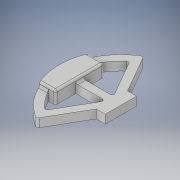
# Autodesk Inventor part: pieceMere
Saved by Autodesk Inventor 2019 (Build 230136000, 136)
## iProperties
Created: 2021-01-08
Part Number: pieceMere
Material: Générique
Document SubType Name: Modeling
Designer: tom.mousset
Density: 1 g/cm^3
Appearance: Par défaut
Author: tom.mousset
Autodesk Inventor part; units mm, degrees
ref_plane "YZ Plane" through (0, 0, 0) normal (1, 0, 0) x (0, 1, 0)
ref_plane "XZ Plane" through (0, 0, 0) normal (0, 1, 0) x (-1, 0, 0)
ref_plane "XY Plane" through (0, 0, 0) normal (0, 0, 1) x (1, 0, 0)
sketch "Esquisse1" plane through (0, 0, 0) normal (0, 1, 0) x (-1, 0, 0)
  circle A0 centre (0, 0) radius 80 construction
  line L0 (0, 0) -> (40, 69.282) construction
  line L1 (0, 0) -> (40, -69.282) construction
  line L2 (0, 0) -> (26.8174, 0)
  line L3 (78.7655, 14) -> (78.7655, 26) construction
  line L4 (78.7655, 26) -> (57.7655, 26) construction
  line L5 (57.7655, 26) -> (57.7655, 14) construction
  line L6 (57.7655, 14) -> (78.7655, 14) construction
  line L7 (78.7655, -14) -> (78.7655, -26) construction
  line L8 (78.7655, -26) -> (57.7655, -26) construction
  line L9 (57.7655, -26) -> (57.7655, -14) construction
  line L10 (57.7655, -14) -> (78.7655, -14) construction
  arc A1 (40, -69.282) -> (40, 69.282) centre (0, 0) ccw construction
  arc A2 (39.5, -68.416) -> (39.5, 68.416) centre (0, 0) ccw construction
  line L11 (0, 20) -> (0, -20)
  line L12 (0, 20) -> (11.547, 20)
  line L13 (0, -20) -> (11.547, -20)
  line L14 (47.8425, -62.8657) -> (11.547, 0) construction
  line L15 (11.547, 0) -> (47.8425, 62.8657) construction
  arc A3 (42.796, -54.1249) -> (42.796, 54.1249) centre (0, 0) ccw construction
  line L16 (61.6441, -31) -> (52.7655, -31)
  line L17 (52.7655, -31) -> (52.7655, -5)
  line L18 (52.7655, 5) -> (52.7655, 31)
  line L19 (52.7655, 31) -> (61.6441, 31)
  arc A4 (67.5648, 14) -> (63.914, 26) centre (0, 0) ccw construction
  arc A5 (63.914, -26) -> (67.5648, -14) centre (0, 0) ccw construction
  arc A6 (42.796, -54.1249) -> (61.6441, -31) centre (0, 0) ccw
  arc A7 (61.6441, 31) -> (42.796, 54.1249) centre (0, 0) ccw
  line L20 (42.796, 54.1249) -> (14.4338, 5)
  line L21 (14.4338, -5) -> (42.796, -54.1249)
  line L22 (52.7655, 5) -> (14.4338, 5)
  line L23 (52.7655, -5) -> (14.4338, -5)
  line L24 (11.547, -20) -> (39.5, -68.416)
  line L25 (11.547, 20) -> (39.5, 68.416)
  arc A8 (74.5989, 26) -> (39.5, 68.416) centre (0, 0) ccw
  arc A9 (77.7496, -14) -> (77.7496, 14) centre (0, 0) ccw
  arc A10 (39.5, -68.416) -> (74.5989, -26) centre (0, 0) ccw
  line L26 (74.5989, -26) -> (57.7655, -26)
  line L27 (57.7655, -14) -> (57.7655, -26)
  line L28 (57.7655, -14) -> (77.7496, -14)
  line L29 (74.5989, 26) -> (57.7655, 26)
  line L30 (57.7655, 26) -> (57.7655, 14)
  line L31 (57.7655, 14) -> (77.7496, 14)
  dimension "d10" = 79
  dimension "d0" = 160
  dimension "d1" = 60
  dimension "d2" = 60
  dimension "d3" = 12
  dimension "d4" = 21
  dimension "d5" = 14
  dimension "d6" = 12
  dimension "d7" = 14
  dimension "d8" = 21
  dimension "d9" = 80
  dimension "d11" = 40
  dimension "d12" = 20
  dimension "d13" = 10
  dimension "d14" = 10
  dimension "d15" = 69
  dimension "d16" = 5
  dimension "d17" = 5
  dimension "d20" = 5
  dimension "d21" = 5
  constraints: 64 end point, 28 point on circle, 17 point on line, 10 centre point, 10 coincident, 9 perpendicular, 8 parallel, 5 collinear, 3 horizontal, 2 vertical, 1 concentric, 11 other
  measures "d0" diameter of A0
  measures "d1" angle of L2 L1
  measures "d2" angle of L2 L0
  measures "d3" distance of L3.start L3.end
  measures "d4" distance of L4.end L3.end
  measures "d5" distance from line of L2.end L6
  measures "d6" distance of L7.start L7.end
  measures "d7" vertical distance of L2.end L7.start
  measures "d8" distance of L7.end L8.end
  measures "d9" radius of A1
  measures "d11" distance of L11.start L11.end
  measures "d12" distance of point (0, 0) L11.start
  measures "d13" distance between parallel lines of L0 L15
  measures "d14" distance between parallel lines of L1 L14
  measures "d15" radius of A3
  measures "d16" distance between parallel lines of L16 L8
  measures "d17" distance between parallel lines of L17 L9
  measures "d20" distance between parallel lines of L5 L18
  measures "d21" distance between parallel lines of L4 L19
extrude "Extrusion1" add sketch "Esquisse1" along normal blind 11
sketch "Esquisse2" plane through (0, 11, 0) normal (0, 1, 0) x (1, 0, 0)
  circle A0 centre (0, 0) radius 79 construction
  line L0 (-52.7655, 31) -> (-61.6441, 31) construction
  line L1 (-61.6441, -31) -> (-52.7655, -31) construction
  line L2 (-52.7655, 31) -> (-52.7655, -31)
  arc A1 (-39.5, 68.416) -> (-74.5989, 26) centre (0, 0) ccw construction
  arc A2 (-74.5989, -26) -> (-39.5, -68.416) centre (0, 0) ccw construction
  arc A3 (-72.6636, 31) -> (-72.6636, -31) centre (0, 0) ccw
  line L3 (-52.7655, 31) -> (-72.6636, 31)
  line L4 (-72.6636, -31) -> (-52.7655, -31)
  constraints: 6 end point, 5 point on circle, 2 centre point, 2 coincident, 2 collinear, 1 perpendicular
extrude "Extrusion2" add sketch "Esquisse2" along normal blind 5
fillet "Congé1" radius 2.5 16 edges at (-67.1539, 11, -31) (-67.1539, 11, 31) (-52.7655, 11, 0) (-62.7145, 16, -31) (-52.7655, 16, 0) (-62.7145, 16, 31) (-52.7655, 5.5, 31) (-52.7655, 13.5, 31) (-52.7655, 5.5, -31) (-52.7655, 13.5, -31) (-42.796, 5.5, -54.1249) (-14.4338, 5.5, -5) (-14.4338, 5.5, 5) (-42.796, 5.5, 54.1249) (-39.5, 5.5, -68.416) (-39.5, 5.5, 68.416)
